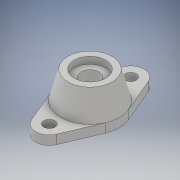
# Autodesk Inventor part: SólidoC
Saved by Autodesk Inventor 2018 (Build 220112000, 112)
## iProperties
Created: 2017-10-07
Part Number: SólidoC
Material: Generic
Document SubType Name: Modeling
Designer: Soichi
Density: 1 g/cm^3
Appearance: Default
Author: Soichi
Autodesk Inventor part; units mm, degrees
ref_plane "YZ Plane" through (0, 0, 0) normal (1, 0, 0) x (0, 1, 0)
ref_plane "XZ Plane" through (0, 0, 0) normal (0, 1, 0) x (-1, 0, 0)
ref_plane "XY Plane" through (0, 0, 0) normal (0, 0, 1) x (1, 0, 0)
sketch "Sketch1" plane through (0, 0, 0) normal (0, 1, 0) x (-1, 0, 0)
  circle A0 centre (0, 0) radius 19.05
  circle A1 centre (0, 0) radius 41.275 construction
  line L0 (0, -57.15) -> (0, 57.15) construction
  circle A2 centre (0, -57.15) radius 7.9375
  line L1 (57.785, 0) -> (-57.785, 0) construction
  circle A3 centre (0, -57.15) radius 19.05 construction
  circle A4 centre (0, 57.15) radius 7.9375
  circle A5 centre (0, 57.15) radius 19.05 construction
  line L2 (-17.5505, -64.5583) -> (-38.026, -16.0514)
  line L3 (17.5505, -64.5583) -> (38.026, -16.0514)
  line L4 (-17.5505, 64.5583) -> (-38.026, 16.0514)
  line L5 (17.5505, 64.5583) -> (38.026, 16.0514)
  arc A6 (-17.5505, -64.5583) -> (17.5505, -64.5583) centre (0, -57.15) ccw
  arc A7 (17.5505, 64.5583) -> (-17.5505, 64.5583) centre (0, 57.15) ccw
  arc A8 (-38.026, 16.0514) -> (-38.026, -16.0514) centre (0, 0) ccw
  arc A9 (38.026, -16.0514) -> (38.026, 16.0514) centre (0, 0) ccw
  dimension "d1" = 82.55
  dimension "d4" = 38.1
  dimension "d0" = 38.1
  dimension "d2" = 114.3
  dimension "d3" = 15.875
  constraints: 10 coincident, 10 end point, 8 centre point, 8 point on circle, 8 symmetric about line, 1 midpoint, 1 vertical, 10 other
  measures "d0" diameter of A0
  measures "d2" distance of L0.start L0.end
  measures "d3" diameter of A2
extrude "Extrusion1" add sketch "Sketch1" along normal blind 12.7
sketch "Sketch2" plane through (0, 0, 0) normal (1, 0, 0) x (0, 1, 0)
  line L0 (0, -19.05) -> (12.7, -19.05) construction
  line L1 (12.7, -19.05) -> (19.05, -19.05)
  line L2 (19.05, -19.05) -> (25.4, -12.7)
  line L3 (25.4, -12.7) -> (41.148, -12.7)
  line L4 (41.148, -12.7) -> (41.148, -22.225)
  line L5 (41.148, -22.225) -> (50.8, -22.225)
  line L6 (50.8, -22.225) -> (50.8, -31.0661)
  line L7 (50.8, -31.0661) -> (12.7, -41.275)
  line L8 (12.7, -64.5583) -> (12.7, -16.0514) construction
  line L9 (0, -16.0514) -> (0, -64.5583) construction
  line L10 (12.7, -19.05) -> (12.7, -41.275)
  line L11 (12.7, -19.05) -> (12.7, -41.275)
  line L12 (12.7, -41.275) -> (50.8, -31.0661)
  line L13 (50.8, -31.0661) -> (50.8, -22.225)
  line L14 (41.148, -22.225) -> (50.8, -22.225)
  line L15 (41.148, -22.225) -> (41.148, -12.7)
  line L16 (41.148, -12.7) -> (25.4, -12.7)
  line L17 (25.4, -12.7) -> (19.05, -19.05)
  line L18 (19.05, -19.05) -> (12.7, -19.05)
  line L19 (12.7, -41.275) -> (28.7707, -41.275) construction
  line L20 (-10.16, 0) -> (60.96, 0) construction
  point P0 (0, 0)
  dimension "d7" = 50.8
  dimension "d8" = 19.05
  dimension "d9" = 12.7
  dimension "d10" = 41.275
  dimension "d12" = 22.225
  dimension "d13" = 9.652
  dimension "d14" = 25.4
  dimension "d16" = 15
  constraints: 34 end point, 9 collinear, 2 horizontal, 2 point on line, 2 vertical, 1 parallel, 1 perpendicular
  measures "d7" distance between parallel lines of L9 L6
  measures "d8" distance from line of L9 L1.end
  measures "d9" distance from line of point (0, 0) L3
  measures "d10" vertical distance of point (0, 0) L7.end
  measures "d12" vertical distance of point (0, 0) L5.end
  measures "d13" distance of L4.end L5.end
  measures "d14" distance from line of L9 L2.end
  measures "d16" angle of L7 L19
revolve "Revolution1" add sketch "Sketch2" angle 360 about axis through (0, -10, 0) along (0, 1, 0)
body "Solid1"
